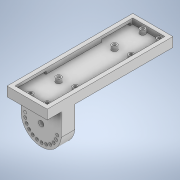
# Autodesk Inventor part: pi_cam_stereo_board
Saved by Autodesk Inventor 2021 (Build 250183000, 183)
## iProperties
Created: 2020-10-30
Part Number: pi_cam_stereo_board
Material: Generic
Document SubType Name: Modeling
Designer: Mateusz
Density: 1 g/cm^3
Appearance: Default
Author: Mateusz
Autodesk Inventor part; units mm, degrees
ref_plane "YZ Plane" through (0, 0, 0) normal (1, 0, 0) x (0, 1, 0)
ref_plane "XZ Plane" through (0, 0, 0) normal (0, 1, 0) x (-1, 0, 0)
ref_plane "XY Plane" through (0, 0, 0) normal (0, 0, 1) x (1, 0, 0)
sketch "Sketch1" plane through (0, 0, 0) normal (0, 1, 0) x (-1, 0, 0)
  line L0 (0, 0) -> (0, -62.5)
  line L1 (9.458, 0) -> (9.458, 12.5)
  line L2 (9.458, 12.5) -> (9.458, -12.5)
  line L3 (9.458, 12.5) -> (-14.404, 12.5)
  line L4 (-14.404, 12.5) -> (-14.404, -12.5)
  line L5 (-14.404, -12.5) -> (9.458, -12.5)
  line L6 (-14.404, 12.5) -> (-12.404, 12.5)
  line L7 (-14.404, -12.5) -> (-12.404, -12.5)
  circle A0 centre (0.096, 10.5) radius 1.1
  circle A1 centre (-12.404, 10.5) radius 1.1
  circle A2 centre (-12.404, -10.5) radius 1.1
  circle A3 centre (0.096, -10.5) radius 1.1
  line L8 (9.458, -62.5) -> (9.458, -50)
  line L9 (9.458, -50) -> (9.458, -75)
  line L10 (9.458, -50) -> (-14.404, -50)
  line L11 (-14.404, -50) -> (-14.404, -75)
  line L12 (-14.404, -75) -> (9.458, -75)
  line L13 (-14.404, -50) -> (-12.404, -50)
  line L14 (-14.404, -75) -> (-12.404, -75)
  circle A4 centre (0.096, -52) radius 1.1
  circle A5 centre (-12.404, -52) radius 1.1
  circle A6 centre (-12.404, -73) radius 1.1
  circle A7 centre (0.096, -73) radius 1.1
  line L15 (12.458, 15.5) -> (-17.404, 15.5)
  line L16 (-17.404, 15.5) -> (-17.404, -78)
  line L17 (-17.404, -78) -> (12.458, -78)
  line L18 (12.458, -78) -> (12.458, 15.5)
  line L19 (-14.404, -12.5) -> (-14.404, -50)
  line L20 (9.458, -50) -> (9.458, -12.5)
  constraints: 42 end point, 8 centre point, 8 perpendicular, 6 point on line, 3 vertical, 2 parallel, 1 collinear, 1 horizontal
extrude "Extrusion1" add sketch "Sketch1" against normal blind 3 contours L5 L4 L3 L1 L2 | L5 L20 L10 L0 | L0 L10 L19 L5 | L10 L8 L9 L12 L11 | L18 L17 L16 L15
sketch "Sketch2" plane through (0, 0, 0) normal (0, 1, 0) x (1, 0, 0)
  circle A0 centre (-0.096, -10.5) radius 1.1 projected
  circle A1 centre (-0.096, -10.5) radius 2
  circle A2 centre (12.404, -10.5) radius 1.1 projected
  circle A3 centre (12.404, -10.5) radius 2
  circle A4 centre (12.404, 10.5) radius 1.1 projected
  circle A5 centre (12.404, 10.5) radius 2
  circle A6 centre (-0.096, 10.5) radius 2
  circle A7 centre (-0.096, 52) radius 1.1 projected
  circle A8 centre (-0.096, 52) radius 2
  circle A9 centre (-0.096, 73) radius 1.1 projected
  circle A10 centre (-0.096, 73) radius 2
  circle A11 centre (12.404, 73) radius 1.1 projected
  circle A12 centre (12.404, 73) radius 2
  circle A13 centre (12.404, 52) radius 1.1 projected
  circle A14 centre (12.404, 52) radius 2
  circle A15 centre (-0.096, 73) radius 1.1
  circle A16 centre (12.404, 73) radius 1.1
  circle A17 centre (12.404, 52) radius 1.1
  circle A18 centre (-0.096, 52) radius 1.1
  circle A19 centre (-0.096, 10.5) radius 1.1
  circle A20 centre (12.404, 10.5) radius 1.1
  circle A21 centre (12.404, -10.5) radius 1.1
  circle A22 centre (-0.096, -10.5) radius 1.1
  circle A23 centre (-0.096, 10.5) radius 1.1
  point P0 (0, 0)
  dimension "d21" = 4
  dimension "d22" = 4
  dimension "d23" = 4
  dimension "d24" = 4
  dimension "d25" = 4
  dimension "d26" = 4
  dimension "d27" = 4
  dimension "d28" = 4
  constraints: 17 centre point, 16 coincident, 8 concentric
  measures "d21" diameter of A1
  measures "d22" diameter of A3
  measures "d23" diameter of A5
  measures "d24" diameter of A6
  measures "d25" diameter of A8
  measures "d26" diameter of A10
  measures "d27" diameter of A12
  measures "d28" diameter of A14
extrude "Extrusion2" add sketch "Sketch2" along normal blind 3
extrude "Extrusion3" add sketch "Sketch1" along normal blind 4 contours L18 L17 L16 L15
sketch "Sketch3" plane through (-12.458, -3, -78) normal (-1, 0, 0) x (0, 0, 1)
  line L0 (89.6, 0) -> (87.4, 0) projected
  line L1 (68.6, 0) -> (66.4, 0) projected
  line L2 (27.1, 0) -> (24.9, 0) projected
  line L3 (6.1, 0) -> (3.9, 0) projected
  line L4 (88.5, 0) -> (88.5, 3)
  line L5 (88.5, 3) -> (88.5, 5)
  line L6 (88.5, 3) -> (88.5, 6) projected
  line L7 (88.5, 5) -> (67.5, 5)
  line L8 (67.5, 3) -> (67.5, 6) projected
  line L9 (67.5, 5) -> (67.5, 3)
  line L10 (67.5, 3) -> (88.5, 3)
  line L11 (27.1, 0) -> (24.9, 0) projected
  line L12 (26, 0) -> (26, 5)
  line L13 (26, 5) -> (5, 5)
  line L14 (5, 3) -> (5, 6) projected
  line L15 (5, 5) -> (5, 3)
  line L16 (26, 3) -> (5, 3) projected
  line L17 (5, 3) -> (26, 3)
  dimension "d33" = 2
  dimension "d34" = 5
  constraints: 18 end point, 6 point on line, 3 perpendicular, 2 midpoint, 1 collinear, 1 vertical
  measures "d33" distance of L4.end L5.end
  measures "d34" distance of L12.start L12.end
extrude "Extrusion4" cut sketch "Sketch3" against normal up to surface (3 mm away)
sketch "Sketch4" plane through (-12.458, -3, -78) normal (-1, 0, 0) x (0, 0, 1)
  line L0 (0, 0) -> (93.5, 0) projected
  line L1 (78, 0) -> (78, -30)
  line L2 (78, -30) -> (83, -30)
  line L3 (83, -30) -> (73, -30)
  line L4 (73, -30) -> (73, 0)
  line L5 (83, -30) -> (83, 0)
  line L6 (73, 0) -> (83, 0)
  line L7 (78, 3) -> (78, -30)
  point P0 (78, -30)
  point P1 (83, 0)
  point P2 (73, 0)
  dimension "d37" = 30
  dimension "d38" = 5
  dimension "d39" = 10
  constraints: 14 end point, 4 perpendicular, 2 vertical, 1 point on line
  measures "d37" distance of L1.start L1.end
  measures "d38" distance of L1.end L2.end
  measures "d39" distance of L2.end L3.end
extrude "Extrusion5" add sketch "Sketch4" against normal up to surface (29.862 mm away)
sketch "Sketch5" plane through (-12.458, -33, 5) normal (0, 0, 1) x (1, 0, 0)
  line L0 (0, 0) -> (29.862, 0) projected
  line L1 (0, 30) -> (0, 0) projected
  circle A0 centre (14.931, 15) radius 15
  line L2 (29.862, 30) -> (29.862, 0) projected
  line L3 (29.862, 0) -> (29.862, 15)
  point P0 (12.458, 33)
  point P1 (29.862, 13.5629)
  point P2 (14.931, 0)
  point P3 (0, 13.5629)
  constraints: 2 end point, 1 centre point, 1 midpoint
extrude "Extrusion6" cut sketch "Sketch5" against normal up to surface (10 mm away) contours L1 A0 L0 | A0 L2 L0
sketch "Sketch6" plane through (-12.458, -3, 5) normal (0, 0, 1) x (1, 0, 0)
  line L0 (29.862, -30) -> (29.862, 0) projected
  line L1 (29.862, -16.4371) -> (26.862, -16.4371)
  circle A0 centre (26.862, -16.4371) radius 1.1
  arc A1 (0, -16.4371) -> (29.862, -16.4371) centre (14.931, -15) ccw projected
  circle A2 centre (14.931, -15) radius 4.093
  circle A3 centre (25.9738, -19.7402) radius 1.1
  circle A4 centre (24.191, -22.6593) radius 1.1
  circle A5 centre (21.6581, -24.9579) radius 1.1
  circle A6 centre (18.5801, -26.4498) radius 1.1
  circle A7 centre (15.2065, -27.0141) radius 1.1
  circle A8 centre (11.8106, -26.605) radius 1.1
  circle A9 centre (8.6675, -25.2558) radius 1.1
  circle A10 centre (6.0318, -23.0758) radius 1.1
  circle A11 centre (4.1171, -20.2414) radius 1.1
  circle A12 centre (3.0784, -16.9825) radius 1.1
  circle A13 centre (3, -13.5629) radius 1.1
  point P0 (12.458, 3)
  dimension "d46" = 3
  dimension "d47" = 2.2
  dimension "d50" = 180
  constraints: 13 centre point, 2 coincident, 2 end point, 1 horizontal, 23 other
  measures "d46" distance of L1.start L1.end
  measures "d47" diameter of A0
extrude "Extrusion7" cut sketch "Sketch6" against normal up to surface (10 mm away) contours A0 | A3 | A4 | A5 | A6 | A7 | A8 | A9 | A10 | A11 | A12 | A13
sketch "Sketch7" plane through (-12.458, -3, 5) normal (0, 0, 1) x (1, 0, 0)
  arc A0 (0, -16.4371) -> (29.862, -16.4371) centre (14.931, -15) ccw projected
  circle A1 centre (14.931, -15) radius 2
  point P0 (12.458, 3)
  dimension "d54" = 4
  constraints: 1 centre point, 1 coincident
  measures "d54" diameter of A1
extrude "Extrusion8" cut sketch "Sketch7" against normal up to surface (10 mm away)
body "Solid1"
